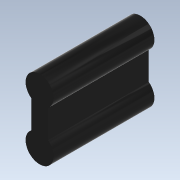
# Autodesk Inventor part: index_joint
Saved by Autodesk Inventor 2020.2 (Build 242310000, 310)
## iProperties
Created: 2020-05-31
Part Number: index_joint
Material: Generic
Document SubType Name: Modeling
Designer: Bardo91
Density: 1 g/cm^3
Appearance: Default
Author: Bardo91
Autodesk Inventor part; units mm, degrees
ref_plane "YZ Plane" through (0, 0, 0) normal (1, 0, 0) x (0, 1, 0)
ref_plane "XZ Plane" through (0, 0, 0) normal (0, 1, 0) x (-1, 0, 0)
ref_plane "XY Plane" through (0, 0, 0) normal (0, 0, 1) x (1, 0, 0)
sketch "Sketch1" plane through (0, 0, 0) normal (0, 0, 1) x (1, 0, 0)
  circle A0 centre (0, 0) radius 2.5
  line L0 (0, 0) -> (0, 18)
  circle A1 centre (0, 18) radius 2.5
  line L1 (1.5, 0) -> (1.5, 18)
  line L2 (-1.5, 0) -> (-1.5, 18)
  point P0 (1.5, 2)
  point P1 (1.5, 16)
  point P2 (-1.5, 16)
  point P3 (-1.5, 2)
  dimension "d0" = 5
  dimension "d1" = 18
  dimension "d2" = 5
  dimension "d3" = 1.5
  dimension "d4" = 1.5
  constraints: 6 end point, 2 centre point, 2 coincident, 2 parallel, 1 vertical
  measures "d0" diameter of A0
  measures "d1" distance of L0.start L0.end
  measures "d2" diameter of A1
  measures "d3" distance between parallel lines of L0 L1
  measures "d4" distance between parallel lines of L0 L2
extrude "Extrusion1" add sketch "Sketch1" along normal blind 18
body "Solid1"
